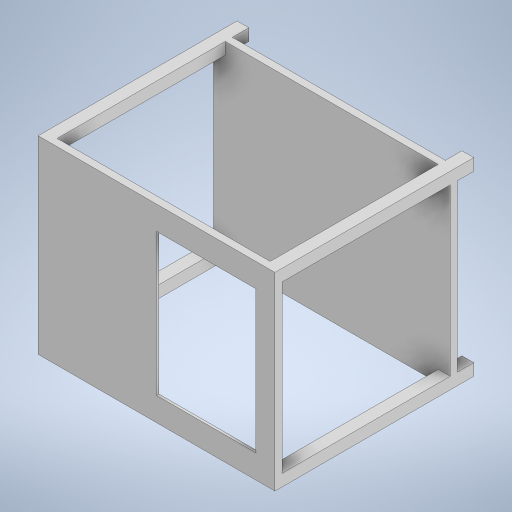
# Autodesk Inventor part: Table
Saved by Autodesk Inventor 2023 (Build 270158000, 158)
## iProperties
Created: 2022-09-30
Part Number: Table
Material: Generic
Document SubType Name: Modeling
Designer: benni
Density: 1 g/cm^3
Appearance: Default
Author: benni
Autodesk Inventor part; units mm, degrees
ref_plane "YZ Plane" through (0, 0, 0) normal (1, 0, 0) x (0, 1, 0)
ref_plane "XZ Plane" through (0, 0, 0) normal (0, 1, 0) x (-1, 0, 0)
sketch "Sketch1" plane through (0, 0, 0) normal (0, 0, 1) x (1, 0, 0)
  line L0 (0, -10) -> (0, 10)
  line L1 (10, 0) -> (-10, 0)
  line L2 (225, 175) -> (250, 175)
  line L3 (250, 175) -> (250, 200)
  line L4 (250, 200) -> (225, 200)
  line L5 (225, 200) -> (225, 175)
  line L6 (-225, 175) -> (-250, 175)
  line L7 (-250, 175) -> (-250, 200)
  line L8 (-250, 200) -> (-225, 200)
  line L9 (-225, 200) -> (-225, 175)
  line L10 (225, -175) -> (250, -175)
  line L11 (250, -175) -> (250, -200)
  line L12 (250, -200) -> (225, -200)
  line L13 (225, -200) -> (225, -175)
  line L14 (-225, -200) -> (-225, -175)
  line L15 (-250, -200) -> (-225, -200)
  line L16 (-250, -175) -> (-250, -200)
  line L17 (-225, -175) -> (-250, -175)
  point P0 (0, 0)
  dimension "d0" = 20
  dimension "d1" = 20
  dimension "d2" = 25
  dimension "d3" = 25
  dimension "d4" = 500
  dimension "d5" = 400
  constraints: 36 end point, 12 symmetric about line, 3 horizontal, 2 parallel, 2 vertical, 1 perpendicular
  measures "d0" distance of L0.start L0.end
  measures "d1" distance of L1.start L1.end
  measures "d2" distance of L4.end L3.end
  measures "d3" distance of L3.end L2.end
  measures "d4" distance between parallel lines of L3 L7
  measures "d5" distance between parallel lines of L12 L4
extrude "Extrusion1" add sketch "Sketch1" along normal blind 420
ref_plane "Work Plane1" through (0, 0, 50) normal (0, 0, 1) x (1, 0, 0)
sketch "Sketch6" plane through (0, 0, 50) normal (0, 0, 1) x (1, 0, 0)
  line L0 (-250, -175) -> (-250, -200) projected
  line L1 (250, 175) -> (250, 200) projected
  line L2 (-250, -200) -> (250, -200)
  line L3 (250, -200) -> (250, 200)
  line L4 (250, 200) -> (-250, 200)
  line L5 (-250, 200) -> (-250, -200)
  point P0 (0, 0)
  constraints: 8 end point, 2 parallel, 1 horizontal, 1 perpendicular
extrude "Extrusion6" add sketch "Sketch6" against normal blind 5
sketch "Sketch7" plane through (0, 0, 45) normal (0, 0, -1) x (-1, 0, 0)
  line L0 (250, -200) -> (225, -200) projected
  line L1 (-250, 200) -> (-225, 200) projected
  line L2 (250, -200) -> (-250, -200)
  line L3 (-250, -200) -> (-250, 200)
  line L4 (-250, 200) -> (250, 200)
  line L5 (250, 200) -> (250, -200)
  line L6 (225, -175) -> (250, -175) projected
  line L7 (-225, 175) -> (-225, 200) projected
  line L8 (225, -175) -> (-225, -175)
  line L9 (-225, -175) -> (-225, 175)
  line L10 (-225, 175) -> (225, 175)
  line L11 (225, 175) -> (225, -175)
  point P0 (0, 0)
  constraints: 16 end point, 4 parallel, 2 horizontal, 2 perpendicular
extrude "Extrusion7" add sketch "Sketch7" along normal blind 10 contours L0 L2 L3 L1 L7 L9 L8 L6 L5 | L6 L11 L10 L7 L4 L5
sketch "Sketch8" plane through (0, 0, 420) normal (0, 0, 1) x (1, 0, 0)
  line L0 (-225, 200) -> (-250, 200) projected
  line L1 (250, -200) -> (250, -175) projected
  line L2 (-250, 200) -> (250, 200)
  line L3 (250, 200) -> (250, -200)
  line L4 (250, -200) -> (-250, -200)
  line L5 (-250, -200) -> (-250, 200)
  line L6 (0, 150) -> (210, 150)
  line L7 (210, 150) -> (210, -150)
  line L8 (210, -150) -> (0, -150)
  line L9 (0, -150) -> (0, 150)
  point P0 (0, 0)
  dimension "d26" = 50
  dimension "d29" = 40
  dimension "d30" = 50
  dimension "d31" = 210
  dimension "d32" = 300
  constraints: 16 end point, 4 parallel, 2 horizontal, 2 perpendicular
  measures "d26" distance between parallel lines of L2 L6
  measures "d29" distance between parallel lines of L3 L7
  measures "d30" distance between parallel lines of L4 L8
  measures "d31" distance between parallel lines of L9 L7
  measures "d32" distance between parallel lines of L8 L6
extrude "Extrusion8" add sketch "Sketch8" against normal blind 5
sketch "Sketch9" plane through (0, 0, 415) normal (0, 0, -1) x (-1, 0, 0)
  line L0 (250, -175) -> (250, -200) projected
  line L1 (-250, 200) -> (-225, 200) projected
  line L2 (250, -200) -> (-250, -200)
  line L3 (-250, -200) -> (-250, 200)
  line L4 (-250, 200) -> (250, 200)
  line L5 (250, 200) -> (250, -200)
  line L6 (225, -175) -> (250, -175) projected
  line L7 (-250, 175) -> (-225, 175) projected
  line L8 (225, -175) -> (-225, -175)
  line L9 (-225, -175) -> (-225, 175)
  line L10 (-225, 175) -> (225, 175)
  line L11 (225, 175) -> (225, -175)
  point P0 (0, 0)
  constraints: 16 end point, 4 parallel, 2 horizontal, 2 perpendicular
extrude "Extrusion9" add sketch "Sketch9" along normal blind 10 contours L6 L11 L10 L7 L3 L1 L4 L5 | L0 L2 L3 L7 L9 L8 L6
equation "\"d30\" = d26"
body "Solid1"
